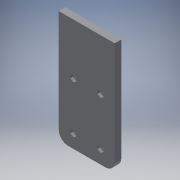
# Autodesk Inventor part: box
Saved by Autodesk Inventor 2017 (Build 210142000, 142)
## iProperties
Created: 2017-09-05
Part Number: box
Material: Generic
Document SubType Name: Modeling
Designer: Hp
Density: 1 g/cm^3
Appearance: Default
Author: Hp
Autodesk Inventor part; units mm, degrees
ref_plane "YZ Plane" through (0, 0, 0) normal (1, 0, 0) x (0, 1, 0)
ref_plane "XZ Plane" through (0, 0, 0) normal (0, 1, 0) x (-1, 0, 0)
ref_plane "XY Plane" through (0, 0, 0) normal (0, 0, 1) x (1, 0, 0)
sketch "Sketch1" plane through (0, 0, 0) normal (0, 0, 1) x (1, 0, 0)
  circle A0 centre (14.4853, 25.4853) radius 1.625 projected
  circle A1 centre (-14.4853, -25.4853) radius 1.625 projected
  circle A2 centre (-14.4853, 25.4853) radius 1.625 projected
  circle A3 centre (14.4853, -25.4853) radius 1.625 projected
  line L0 (10, 17) -> (10, -17) projected
  arc A4 (6, -21) -> (10, -17) centre (6, -17) ccw projected
  line L1 (6, -21) -> (-6, -21) projected
  arc A5 (-10, -17) -> (-6, -21) centre (-6, -17) ccw projected
  line L2 (-10, -17) -> (-10, 17) projected
  arc A6 (-6, 21) -> (-10, 17) centre (-6, 17) ccw projected
  line L3 (-6, 21) -> (6, 21) projected
  arc A7 (10, 17) -> (6, 21) centre (6, 17) ccw projected
  line L4 (-23, 17) -> (-23, -17) projected
  arc A8 (-23, -17) -> (-6, -34) centre (-6, -17) ccw projected
  line L5 (-6, -34) -> (6, -34) projected
  arc A9 (6, -34) -> (23, -17) centre (6, -17) ccw projected
  line L6 (23, -17) -> (23, 17) projected
  arc A10 (23, 17) -> (6, 34) centre (6, 17) ccw projected
  line L7 (6, 34) -> (-6, 34) projected
  arc A11 (-6, 34) -> (-23, 17) centre (-6, 17) ccw projected
  line L8 (-22, 17) -> (-22, -17)
  arc A12 (-22, -17) -> (-6, -33) centre (-6, -17) ccw
  line L9 (-6, -33) -> (6, -33)
  arc A13 (6, -33) -> (22, -17) centre (6, -17) ccw
  line L10 (22, -17) -> (22, 17)
  arc A14 (22, 17) -> (6, 33) centre (6, 17) ccw
  line L11 (6, 33) -> (-6, 33)
  arc A15 (-6, 33) -> (-22, 17) centre (-6, 17) ccw
  line L12 (-30, 80) -> (30, 80)
  line L13 (30, 80) -> (30, -30)
  line L14 (20, -40) -> (-20, -40)
  line L15 (-30, -30) -> (-30, 80)
  line L16 (0, 0) -> (-30, 0) construction
  line L17 (0, 0) -> (30, 0) construction
  arc A16 (-30, -30) -> (-20, -40) centre (-20, -30) ccw
  arc A17 (20, -40) -> (30, -30) centre (20, -30) ccw
  line L18 (-11.3603, 23.6811) -> (-14.4853, 21.8768)
  line L19 (-14.4853, 21.8768) -> (-17.6103, 23.6811)
  line L20 (-17.6103, 23.6811) -> (-17.6103, 27.2895)
  line L21 (-17.6103, 27.2895) -> (-14.4853, 29.0937)
  line L22 (-14.4853, 29.0937) -> (-11.3603, 27.2895)
  line L23 (-11.3603, 27.2895) -> (-11.3603, 23.6811)
  line L24 (17.6103, -27.2895) -> (14.4853, -29.0937)
  line L25 (14.4853, -29.0937) -> (11.3603, -27.2895)
  line L26 (11.3603, -27.2895) -> (11.3603, -23.6811)
  line L27 (11.3603, -23.6811) -> (14.4853, -21.8768)
  line L28 (14.4853, -21.8768) -> (17.6103, -23.6811)
  line L29 (17.6103, -23.6811) -> (17.6103, -27.2895)
  line L30 (-11.3603, -27.2895) -> (-14.4853, -29.0937)
  line L31 (-14.4853, -29.0937) -> (-17.6103, -27.2895)
  line L32 (-17.6103, -27.2895) -> (-17.6103, -23.6811)
  line L33 (-17.6103, -23.6811) -> (-14.4853, -21.8768)
  line L34 (-14.4853, -21.8768) -> (-11.3603, -23.6811)
  line L35 (-11.3603, -23.6811) -> (-11.3603, -27.2895)
  line L36 (17.6103, 23.6811) -> (14.4853, 21.8768)
  line L37 (14.4853, 21.8768) -> (11.3603, 23.6811)
  line L38 (11.3603, 23.6811) -> (11.3603, 27.2895)
  line L39 (11.3603, 27.2895) -> (14.4853, 29.0937)
  line L40 (14.4853, 29.0937) -> (17.6103, 27.2895)
  line L41 (17.6103, 27.2895) -> (17.6103, 23.6811)
  point P0 (30, -40)
  point P1 (-14.4853, 25.4853)
  point P2 (14.4853, -25.4853)
  point P3 (-14.4853, -25.4853)
  point P4 (14.4853, 25.4853)
  dimension "d0" = 1
  dimension "d1" = 60
  dimension "d2" = 120
  dimension "d4" = 40
  dimension "d5" = 10
  dimension "d6" = 6.25
  dimension "d7" = 6.25
  dimension "d8" = 6.25
  dimension "d9" = 6.25
  constraints: 68 end point, 12 point on circle, 6 centre point, 5 point on line, 4 coincident, 4 tangent, 4 vertical, 2 horizontal, 2 parallel, 1 collinear, 1 equal radius, 1 perpendicular, 59 other
  measures "d0" radial gap between concentric circles of A11 A15
  measures "d1" distance of L12.start L12.end
  measures "d2" distance of L12.end point (30, -40)
  measures "d4" distance from line of L14 L16.start
  measures "d5" radius of A16
  measures "d6" distance between parallel lines of L23 L20
  measures "d7" distance between parallel lines of L29 L26
  measures "d8" distance between parallel lines of L35 L32
  measures "d9" distance between parallel lines of L41 L38
extrude "Extrusion1" add sketch "Sketch1" along normal blind 7 contours A0 | A1 | A2 | A3 | L0 A4 L1 A5 L2 A6 L3 A7 | A11 L7 A10 L6 A9 L5 A8 L4 | A15 L11 A14 L10 A13 L9 A12 L8 | L12 L13 A17 L14 A16 L15 | L18 L19 L20 L21 L22 L23 | L24 L25 L26 L27 L28 L29 | L30 L31 L32 L33 L34 L35 | L36 L37 L38 L39 L40 L41
extrude "Extrusion2" cut sketch "Sketch1" along normal blind 3.5 contours A0 | A1 | A2 | A3 | A15 L11 A14 L10 A13 L9 A12 L8 | L18 L19 L20 L21 L22 L23 | L24 L25 L26 L27 L28 L29 | L30 L31 L32 L33 L34 L35 | L36 L37 L38 L39 L40 L41
sketch "Sketch3" plane through (0, 0, 7) normal (0, 0, 1) x (1, 0, 0)
  line L0 (17.6103, -23.6811) -> (17.6103, -27.2895) projected
  line L1 (17.6103, -27.2895) -> (14.4853, -29.0937) projected
  line L2 (14.4853, -29.0937) -> (11.3603, -27.2895) projected
  line L3 (11.3603, -27.2895) -> (11.3603, -23.6811) projected
  line L4 (11.3603, -23.6811) -> (14.4853, -21.8768) projected
  line L5 (14.4853, -21.8768) -> (17.6103, -23.6811) projected
  circle A0 centre (14.4853, -25.4853) radius 1.625 projected
  line L6 (17.6103, 23.6811) -> (14.4853, 21.8768) projected
  line L7 (17.6103, 27.2895) -> (17.6103, 23.6811) projected
  line L8 (14.4853, 29.0937) -> (17.6103, 27.2895) projected
  line L9 (11.3603, 27.2895) -> (14.4853, 29.0937) projected
  line L10 (11.3603, 23.6811) -> (11.3603, 27.2895) projected
  line L11 (14.4853, 21.8768) -> (11.3603, 23.6811) projected
  circle A1 centre (14.4853, 25.4853) radius 1.625 projected
  line L12 (-11.3603, 23.6811) -> (-14.4853, 21.8768) projected
  line L13 (-14.4853, 21.8768) -> (-17.6103, 23.6811) projected
  line L14 (-11.3603, 27.2895) -> (-11.3603, 23.6811) projected
  line L15 (-14.4853, 29.0937) -> (-11.3603, 27.2895) projected
  line L16 (-17.6103, 27.2895) -> (-14.4853, 29.0937) projected
  line L17 (-17.6103, 23.6811) -> (-17.6103, 27.2895) projected
  circle A2 centre (-14.4853, 25.4853) radius 1.625 projected
  line L18 (-11.3603, -27.2895) -> (-14.4853, -29.0937) projected
  line L19 (-11.3603, -23.6811) -> (-11.3603, -27.2895) projected
  line L20 (-14.4853, -21.8768) -> (-11.3603, -23.6811) projected
  line L21 (-17.6103, -23.6811) -> (-14.4853, -21.8768) projected
  line L22 (-17.6103, -27.2895) -> (-17.6103, -23.6811) projected
  line L23 (-14.4853, -29.0937) -> (-17.6103, -27.2895) projected
  circle A3 centre (-14.4853, -25.4853) radius 1.625 projected
  point P0 (0, 0)
  point P1 (14.4853, -25.4853)
  point P2 (14.4853, 25.4853)
extrude "Extrusion3" cut sketch "Sketch3" against normal blind 3
extrude "Extrusion4" cut sketch "Sketch3" against normal through all contours A0 | A1 | A2 | A3
body "Solid1"
